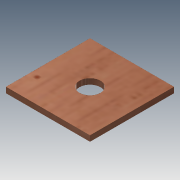
# Autodesk Inventor part: gabarito-30
Saved by Autodesk Inventor 2017 (Build 210142000, 142)
## iProperties
Created: 2018-08-18
Part Number: gabarito-30
Material: Wood (Oak)
Document SubType Name: Sheet Metal
Designer: Luiz Gustavo
Density: 0.76 g/cm^3
Sheet Metal Rule: Default_mm
Appearance: White Oak - Natural Medium Gloss
Author: Luiz Gustavo
Autodesk Inventor part; units mm, degrees
ref_plane "YZ Plane" through (0, 0, 0) normal (1, 0, 0) x (0, 1, 0)
ref_plane "XZ Plane" through (0, 0, 0) normal (0, 1, 0) x (-1, 0, 0)
ref_plane "XY Plane" through (0, 0, 0) normal (0, 0, 1) x (1, 0, 0)
sketch "Sketch1" plane through (0, 0, 0) normal (0, 0, 1) x (1, 0, 0)
  arc A0 (-5.9942, 51.8019) -> (-3.0058, 51.8019) centre (-4.5, 55) ccw
  line L0 (8.4999, 69.9999) -> (0, 69.9999)
  line L1 (-9, 40.0001) -> (-17.4999, 40.0001)
  line L2 (10.4999, 0) -> (10.4999, 69.9999)
  line L3 (-19.4999, 0) -> (-19.4999, 69.9999)
  line L4 (-19.4999, 69.9999) -> (10.4999, 69.9999)
  line L5 (10.4999, 69.9999) -> (10.4999, 40.0001)
  line L6 (10.4999, 40.0001) -> (-19.4999, 40.0001)
  line L7 (-19.4999, 40.0001) -> (-19.4999, 69.9999)
  circle A1 centre (-4.5, 55) radius 3.75
  point P0 (0, 0)
  dimension "d0" = 29.9999
  dimension "d1" = 29.9999
  dimension "d2" = 14.9999
  dimension "d3" = 7.5
  measures "d0" distance between parallel lines of L3 L2
  measures "d1" distance between parallel lines of L1 L0
  measures "d2" distance from line of L0 A0.centre
  measures "d3" diameter of A1
extrude "Plate1" add sketch "Sketch1" along normal blind 2
equation "\"BendRadius\" = Thickness"
equation "\"BendReliefWidth\" = Thickness"
equation "\"BendReliefDepth\" = 0.5 * Thickness"
equation "\"CornerReliefSize\" = 4 * Thickness"
equation "\"MinimumRemnant\" = 2 * Thickness"
equation "\"TransitionRadius\" = BendRadius"
equation "\"JacobiRadiusSize\" = BendRadius"
equation "\"GapSize\" = Thickness"
equation "\"d4\" = BendRadius"
equation "\"Thickness\" = 2"
body "Solid1"
